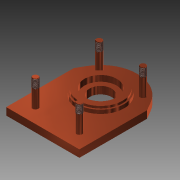
# Autodesk Inventor part: 刀轴端盖
Saved by Autodesk Inventor 2015 (Build 190159000, 159)
## iProperties
Created: 2017-05-17
Part Number: 刀轴端盖
Material: 常规
Document SubType Name: Modeling
Designer: Administrator
Density: 1 g/cm^3
Appearance: 铜 - 抛光
Author: Administrator
Autodesk Inventor part; units mm, degrees
ref_plane "YZ Plane" through (0, 0, 0) normal (1, 0, 0) x (0, 1, 0)
ref_plane "XZ Plane" through (0, 0, 0) normal (0, 1, 0) x (-1, 0, 0)
ref_plane "XY Plane" through (0, 0, 0) normal (0, 0, 1) x (1, 0, 0)
sketch "草图1" plane through (0, 0, 0) normal (0, 0, 1) x (1, 0, 0)
  circle A0 centre (0, 39.5) radius 25
  line L0 (-25, 46.1987) -> (-25, 0)
  line L1 (-25, 0) -> (25, 0)
  line L2 (25, 0) -> (25, 46.1987)
  line L3 (-21.6506, 52) -> (-51.6728, 0)
  line L4 (21.6506, 52) -> (51.6728, 0)
  line L5 (0, 0) -> (0, -13.7014)
  dimension "d0" = 50
  dimension "d1" = 39.5
  dimension "d2" = 13.7014
  dimension "d3" = 60
  constraints: 12 end point, 5 point on line, 4 tangent, 2 perpendicular, 2 point on circle, 2 vertical, 1 centre point, 1 equal length, 1 midpoint
  measures "d0" diameter of A0
  measures "d1" distance of L5.start A0.centre
  measures "d2" distance of L5.start L5.end
  measures "d3" angle of L1 L4
extrude "拉伸1" add sketch "草图1" along normal blind 5
sketch "草图2" plane through (0, 0, 5) normal (0, 0, 1) x (1, 0, 0)
  circle A0 centre (0, 39.5) radius 16
  circle A1 centre (0, 39.5) radius 11
  arc A2 (21.6506, 52) -> (-21.6506, 52) centre (0, 39.5) ccw projected
  point P0 (0, 0)
  dimension "d6" = 32
  dimension "d7" = 22
  constraints: 2 centre point, 1 coincident, 1 concentric
  measures "d6" diameter of A0
  measures "d7" diameter of A1
extrude "拉伸2" add sketch "草图2" along normal blind 4
sketch "草图3" plane through (0, 39.5, 9) normal (0, 0, 1) x (1, 0, 0)
  circle A0 centre (0, 0) radius 16
  circle A1 centre (0, 0) radius 15
  circle A2 centre (0, 0) radius 11 projected
  point P0 (0, -39.5)
  dimension "d10" = 32
  dimension "d11" = 30
  constraints: 2 centre point, 1 coincident, 1 concentric
  measures "d10" diameter of A0
  measures "d11" diameter of A1
extrude "拉伸3" cut sketch "草图3" against normal blind 1.5 contours A0
sketch "草图4" plane through (0, 39.5, 5) normal (0, 0, 1) x (1, 0, 0)
  circle A0 centre (0, 0) radius 7.5
  circle A1 centre (0, 0) radius 11 projected
  point P0 (0, -39.5)
  dimension "d14" = 15
  constraints: 1 centre point, 1 concentric
  measures "d14" diameter of A0
extrude "拉伸4" cut sketch "草图4" against normal through all contours A0
sketch "草图5" plane through (0, 0, 5) normal (0, 0, 1) x (1, 0, 0)
  circle A0 centre (15, 10) radius 2
  circle A1 centre (-15, 10) radius 2
  circle A2 centre (15, 53.4732) radius 2
  circle A3 centre (-15, 53.4732) radius 2
  line L0 (25, 0) -> (25, 46.1987) projected
  line L1 (-25, 0) -> (25, 0) projected
  line L2 (-25, 46.1987) -> (-25, 0) projected
  arc A4 (15, 53.4732) -> (-15, 53.4732) centre (0, 39.5) ccw
  circle A5 centre (0, 39.5) radius 7.5 projected
  point P0 (0, 0)
  dimension "d17" = 4
  dimension "d18" = 4
  dimension "d19" = 4
  dimension "d20" = 4
  dimension "d21" = 10
  dimension "d22" = 10
  dimension "d23" = 10
  dimension "d24" = 10
  dimension "d25" = 20.5
  dimension "d26" = 10
  dimension "d27" = 10
  constraints: 5 centre point, 2 point on circle, 1 concentric
  measures "d17" diameter of A0
  measures "d18" diameter of A1
  measures "d19" diameter of A2
  measures "d20" diameter of A3
  measures "d21" distance from line of L0 A0.centre
  measures "d22" distance from line of L1 A0.centre
  measures "d23" distance from line of L2 A1.centre
  measures "d24" distance from line of A1.centre L1
  measures "d25" radius of A4
  measures "d26" distance from line of L0 A2.centre
  measures "d27" distance from line of L2 A3.centre
extrude "拉伸5" add sketch "草图5" along normal blind 18 contours A0 | A1 | A2 | A3
thread "螺纹1" size "M4x0.7" class "6g" standard "ANSI Metric M Profile" length 6
thread "螺纹2" size "M4x0.7" class "6g" standard "ANSI Metric M Profile" length 6
thread "螺纹3" size "M4x0.7" class "6g" standard "ANSI Metric M Profile" length 6
thread "螺纹4" size "M4x0.7" class "6g" standard "ANSI Metric M Profile" length 6
chamfer "倒角1" distance 0.25 angle 45 4 edges at (-17, 53.4732, 23) (13, 53.4732, 23) (13, 10, 23) (-17, 10, 23)
